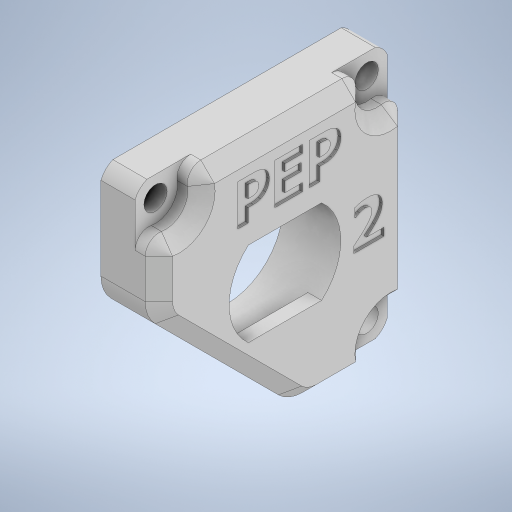
# Autodesk Inventor part: X-Axis-Motor-Support v0.1
Saved by Autodesk Inventor 2023 (Build 270158000, 158)
## iProperties
Created: 2023-07-26
Part Number: X-Axis-Motor-Support v0.1
Material: Generic
Document SubType Name: Modeling
Designer: Parker
Density: 1 g/cm^3
Appearance: Default
Author: Parker
Autodesk Inventor part; units mm, degrees
ref_plane "YZ Plane" through (0, 0, 0) normal (1, 0, 0) x (0, 1, 0)
ref_plane "XZ Plane" through (0, 0, 0) normal (0, 1, 0) x (-1, 0, 0)
ref_plane "XY Plane" through (0, 0, 0) normal (0, 0, 1) x (1, 0, 0)
sketch "Sketch1" plane through (0, 0, 0) normal (1, 0, 0) x (0, 1, 0)
  circle A0 centre (0, 0) radius 8 construction
  circle A1 centre (0, 0) radius 8.2
  line L0 (-15.5, 15.5) -> (15.5, 15.5) construction
  line L1 (15.5, 15.5) -> (15.5, -15.5) construction
  line L2 (15.5, -15.5) -> (-15.5, -15.5) construction
  line L3 (-15.5, -15.5) -> (-15.5, 15.5) construction
  line L4 (-15.5, 15.5) -> (15.5, -15.5) construction
  line L5 (15.5, 15.5) -> (-15.5, -15.5) construction
  line L6 (-18.5, 18.5) -> (18.5, 18.5)
  line L7 (18.5, 18.5) -> (18.5, -18.5)
  line L8 (18.5, -18.5) -> (-18.5, -18.5)
  line L9 (-18.5, -18.5) -> (-18.5, 18.5)
  line L10 (-18.5, 18.5) -> (18.5, -18.5) construction
  line L11 (18.5, 18.5) -> (-18.5, -18.5) construction
  line L12 (-18.5, -2.5) -> (2.5, 18.5)
  point P0 (-15.5, -15.5)
  dimension "d0" = 16
  dimension "d1" = 0.2
  dimension "d2" = 31
  dimension "d3" = 31
  dimension "d4" = 3
  dimension "d5" = 3
  dimension "d6" = 16
  constraints: 26 end point, 5 coincident, 5 parallel, 4 midpoint, 2 centre point, 2 horizontal, 2 perpendicular, 2 point on line
  measures "d0" diameter of A0
  measures "d1" radial gap between concentric circles of A0 A1
  measures "d2" distance of L0.end L1.end
  measures "d3" distance of L0.start L0.end
  measures "d4" distance from line of L8 L1.end
  measures "d5" distance between parallel lines of L7 L1
  measures "d6" distance of L6.end L12.end
extrude "Extrusion1" add sketch "Sketch1" along normal blind 6.5 contours L6 L7 L8 L9 L12
sketch "Sketch2" plane through (6.5, 0, 0) normal (1, 0, 0) x (0, 0, -1)
  point P0 (0, 0)
  point P1 (-15.5, 15.5)
  point P2 (15.5, 15.5)
  point P3 (15.5, -15.5)
hole "Hole1" at (6.5, 15.5, 15.5) at (6.5, 15.5, -15.5) at (6.5, -15.5, -15.5) direction (-1, 0, 0) diameter 3.4 end through all counterbore diameter 6.5 counterbore depth 1.5 clearance for "Socket Head Cap Screw" size "M3" standard "Ansi Metric M Profile"
sketch "Sketch3" plane through (6.5, 0, 0) normal (1, 0, 0) x (0, 0, -1)
  arc A0 (-16.75, 18.5) -> (-18.5, 16.75) centre (-15.5, 15.5) ccw projected
  line L0 (-16.75, 18.5) -> (-18.5, 18.5) projected
  line L1 (-18.5, 18.5) -> (-18.5, 16.75) projected
  arc A1 (18.5, 16.75) -> (16.75, 18.5) centre (15.5, 15.5) ccw projected
  line L2 (18.5, 16.75) -> (18.5, 18.5) projected
  line L3 (18.5, 18.5) -> (16.75, 18.5) projected
  arc A2 (16.75, -18.5) -> (18.5, -16.75) centre (15.5, -15.5) ccw projected
  line L4 (16.75, -18.5) -> (18.5, -18.5) projected
  line L5 (18.5, -18.5) -> (18.5, -16.75) projected
  point P0 (0, 0)
extrude "Extrusion2" cut sketch "Sketch3" against normal through all
fillet "Fillet1" radius 2 6 edges at (5.75, 14.25, 18.5) (5.75, 18.5, 14.25) (5.75, 18.5, -14.25) (5.75, 14.25, -18.5) (5.75, -14.25, -18.5) (5.75, -18.5, -14.25)
fillet "Fillet2" radius 5 2 edges at (3.25, 2.5, 18.5) (3.25, -18.5, -2.5)
sketch "Sketch4" plane through (6.5, 0, 0) normal (1, 0, 0) x (0, 0, -1)
  circle A0 centre (0, 0) radius 8.2 projected
  arc A1 (1.0355, -17.0355) -> (4.5711, -18.5) centre (4.5711, -13.5) ccw projected
  line L0 (4.5711, -18.5) -> (10.3461, -18.5) projected
  arc A2 (10.3461, -18.5) -> (12.3095, -16.119) centre (10.3461, -16.5) ccw projected
  arc A3 (16.119, -12.3095) -> (12.3095, -16.119) centre (15.5, -15.5) ccw projected
  arc A4 (16.119, -12.3095) -> (18.5, -10.3461) centre (16.5, -10.3461) ccw projected
  line L1 (18.5, -10.3461) -> (18.5, 10.3461) projected
  arc A5 (18.5, 10.3461) -> (16.119, 12.3095) centre (16.5, 10.3461) ccw projected
  arc A6 (12.3095, 16.119) -> (16.119, 12.3095) centre (15.5, 15.5) ccw projected
  arc A7 (12.3095, 16.119) -> (10.3461, 18.5) centre (10.3461, 16.5) ccw projected
  line L2 (10.3461, 18.5) -> (-10.3461, 18.5) projected
  arc A8 (-10.3461, 18.5) -> (-12.3095, 16.119) centre (-10.3461, 16.5) ccw projected
  arc A9 (-16.119, 12.3095) -> (-12.3095, 16.119) centre (-15.5, 15.5) ccw projected
  arc A10 (-16.119, 12.3095) -> (-18.5, 10.3461) centre (-16.5, 10.3461) ccw projected
  line L3 (-18.5, 10.3461) -> (-18.5, 4.5711) projected
  arc A11 (-18.5, 4.5711) -> (-17.0355, 1.0355) centre (-13.5, 4.5711) ccw projected
  line L4 (-17.0355, 1.0355) -> (1.0355, -17.0355) projected
  line L5 (-7.5, 10.2) -> (7.5, 10.2)
  line L6 (7.5, 10.2) -> (7.5, 6.2)
  line L7 (7.5, 6.2) -> (-7.5, 6.2)
  line L8 (-7.5, 6.2) -> (-7.5, 10.2)
  circle A12 centre (0, 0) radius 8.2 projected
  line L9 (-7.5, 10.2) -> (7.5, 6.2) construction
  line L10 (7.5, 10.2) -> (-7.5, 6.2) construction
  line L11 (-7.5, -6.2) -> (7.5, -6.2)
  line L12 (7.5, -6.2) -> (7.5, -10.2)
  line L13 (7.5, -10.2) -> (-7.5, -10.2)
  line L14 (-7.5, -10.2) -> (-7.5, -6.2)
  line L15 (-7.5, -6.2) -> (7.5, -10.2) construction
  line L16 (7.5, -6.2) -> (-7.5, -10.2) construction
  point P0 (0, 8.2)
  point P1 (0, -8.2)
  point P2 (-7.5, -8.5)
  point P3 (-5.8, -10.2)
  point P4 (-5.3666, -6.2)
  point P5 (-5.3666, 6.2)
  point P6 (5.3666, 6.2)
  point P7 (5.3666, -6.2)
  dimension "d20" = 15
  dimension "d21" = 4
  dimension "d22" = 15
  dimension "d23" = 4
  constraints: 24 end point, 4 midpoint, 4 parallel, 2 horizontal, 2 perpendicular, 2 point on circle
  measures "d20" distance of L6.end L7.end
  measures "d21" distance of L5.end L6.end
  measures "d22" distance of L12.end L13.end
  measures "d23" distance of L11.end L12.end
extrude "Extrusion3" add sketch "Sketch4" along normal blind 2 contours A0 L7 L6 L5 L8 L11 L14 L4 A11 L3 A10 A9 A8 L2 A7 A6 A5 L1 A4 A3 A2 L0 A1 L13 L12 | L7 A0 | A0 L7 L8 L5 L6 | L11 L12 L13 L4 L14 A0 | A0 L11
chamfer "Chamfer2" distance 2 angle 45 16 edges at (8.5, 18.5, 0) (8.5, 17.7724, 11.8892) (8.5, 13.2019, 13.2019) (8.5, 11.8892, 17.7724) (8.5, 7.4586, 18.5) (8.5, 2.6577, 18.1194) (8.5, -8, 8) (8.5, -18.1194, -2.6577) (8.5, -18.5, -7.4586) (8.5, -17.7724, -11.8892) (8.5, -13.2019, -13.2019) (8.5, -11.8892, -17.7724) (8.5, 0, -18.5) (8.5, 11.8892, -17.7724) (8.5, 13.2019, -13.2019) (8.5, 17.7724, -11.8892)
sketch "Sketch5" plane through (8.5, 0, 0) normal (1, 0, 0) x (0, 0, -1)
  line L0 (9.5104, 3.5032) -> (16.5185, 3.5032) construction
  line L1 (16.5185, 3.5032) -> (16.5185, -4.6524) construction
  line L2 (16.5185, -4.6524) -> (9.5104, -4.6524) construction
  line L3 (9.5104, -4.6524) -> (9.5104, 3.5032) construction
  line L4 (-7.5472, 15.0221) -> (-0.5391, 15.0221) construction
  line L5 (-0.5391, 15.0221) -> (-0.5391, 6.8665) construction
  line L6 (-0.5391, 6.8665) -> (-7.5472, 6.8665) construction
  line L7 (-7.5472, 6.8665) -> (-7.5472, 15.0221) construction
  line L8 (14.5282, -2.6135) -> (10.1182, -2.6135)
  line L9 (10.1182, -2.6135) -> (10.1182, -1.6362)
  spline S0 degree 2 poles (10.1182, -1.6362) (10.6773, -1.1889) (11.572, -0.4012) (11.9075, -0.0463) knots 0 0 0 1 2 2 2
  spline S1 degree 2 poles (11.9075, -0.0463) (12.3499, 0.4156) (12.7438, 1.1207) (12.7438, 1.4902) knots 0 0 0 1 2 2 2
  spline S2 degree 2 poles (12.7438, 1.4902) (12.7438, 1.9083) (12.243, 2.3557) (11.7956, 2.3557) knots 0 0 0 1 2 2 2
  spline S3 degree 2 poles (11.7956, 2.3557) (11.5671, 2.3557) (11.1587, 2.2438) (10.9496, 2.1563) knots 0 0 0 1 2 2 2
  spline S4 degree 2 poles (10.9496, 2.1563) (10.7454, 2.0639) (10.4537, 1.8694) (10.3807, 1.8208) knots 0 0 0 1 2 2 2
  line L10 (10.3807, 1.8208) -> (10.264, 1.8208)
  line L11 (10.264, 1.8208) -> (10.264, 3.1288)
  spline S5 degree 2 poles (10.264, 3.1288) (10.5169, 3.2503) (11.5963, 3.5032) (12.0971, 3.5032) knots 0 0 0 1 2 2 2
  spline S6 degree 2 poles (12.0971, 3.5032) (13.1668, 3.5032) (14.2656, 2.5502) (14.2656, 1.6895) knots 0 0 0 1 2 2 2
  spline S7 degree 2 poles (14.2656, 1.6895) (14.2656, 1.1596) (13.7648, 0.1385) (13.1862, -0.445) knots 0 0 0 1 2 2 2
  spline S8 degree 2 poles (13.1862, -0.445) (12.8216, -0.8048) (12.136, -1.3639) (11.9853, -1.4806) knots 0 0 0 1 2 2 2
  line L12 (11.9853, -1.4806) -> (14.5282, -1.4806)
  line L13 (14.5282, -1.4806) -> (14.5282, -2.6135)
  spline S9 degree 2 poles (-2.3106, 13.1307) (-2.3106, 12.7126) (-2.578, 11.9541) (-2.826, 11.7012) knots 0 0 0 1 2 2 2
  spline S10 degree 2 poles (-2.826, 11.7012) (-2.9767, 11.5408) (-3.3462, 11.2782) (-3.565, 11.1858) knots 0 0 0 1 2 2 2
  spline S11 degree 2 poles (-3.565, 11.1858) (-3.7887, 11.0935) (-4.309, 10.9865) (-4.6299, 10.9865) knots 0 0 0 1 2 2 2
  line L14 (-4.6299, 10.9865) -> (-5.4176, 10.9865)
  line L15 (-5.4176, 10.9865) -> (-5.4176, 9.0221)
  line L16 (-5.4176, 9.0221) -> (-6.9249, 9.0221)
  line L17 (-6.9249, 9.0221) -> (-6.9249, 15.0221)
  line L18 (-6.9249, 15.0221) -> (-4.5958, 15.0221)
  spline S12 degree 2 poles (-4.5958, 15.0221) (-4.0804, 15.0221) (-3.3268, 14.8325) (-3.0205, 14.6283) knots 0 0 0 1 2 2 2
  spline S13 degree 2 poles (-3.0205, 14.6283) (-2.6801, 14.3998) (-2.3106, 13.651) (-2.3106, 13.1307) knots 0 0 0 1 2 2 2
  spline S14 degree 2 poles (-3.8568, 13.0918) (-3.8568, 13.3495) (-4.0999, 13.7142) (-4.2652, 13.7823) knots 0 0 0 1 2 2 2
  spline S15 degree 2 poles (-4.2652, 13.7823) (-4.4791, 13.8747) (-4.8681, 13.9038) (-5.2036, 13.9038) knots 0 0 0 1 2 2 2
  line L19 (-5.2036, 13.9038) -> (-5.4176, 13.9038)
  line L20 (-5.4176, 13.9038) -> (-5.4176, 12.1048)
  line L21 (-5.4176, 12.1048) -> (-5.3106, 12.1048)
  spline S16 degree 2 poles (-5.3106, 12.1048) (-5.1015, 12.1048) (-4.7223, 12.1145) (-4.5813, 12.1388) knots 0 0 0 1 2 2 2
  spline S17 degree 2 poles (-4.5813, 12.1388) (-4.4597, 12.1583) (-4.1923, 12.275) (-4.1193, 12.3479) knots 0 0 0 1 2 2 2
  spline S18 degree 2 poles (-4.1193, 12.3479) (-3.9637, 12.4938) (-3.8568, 12.8195) (-3.8568, 13.0918) knots 0 0 0 1 2 2 2
  line L22 (-1.5035, 9.0221) -> (-1.5035, 15.0221)
  line L23 (-1.5035, 15.0221) -> (2.5516, 15.0221)
  line L24 (2.5516, 15.0221) -> (2.5516, 13.8795)
  line L25 (2.5516, 13.8795) -> (-0.0059, 13.8795)
  line L26 (-0.0059, 13.8795) -> (-0.0059, 12.8244)
  line L27 (-0.0059, 12.8244) -> (2.3523, 12.8244)
  line L28 (2.3523, 12.8244) -> (2.3523, 11.6818)
  line L29 (2.3523, 11.6818) -> (-0.0059, 11.6818)
  line L30 (-0.0059, 11.6818) -> (-0.0059, 10.1648)
  line L31 (-0.0059, 10.1648) -> (2.5516, 10.1648)
  line L32 (2.5516, 10.1648) -> (2.5516, 9.0221)
  line L33 (2.5516, 9.0221) -> (-1.5035, 9.0221)
  spline S19 degree 2 poles (8.187, 13.1307) (8.187, 12.7126) (7.9196, 11.9541) (7.6716, 11.7012) knots 0 0 0 1 2 2 2
  spline S20 degree 2 poles (7.6716, 11.7012) (7.5209, 11.5408) (7.1513, 11.2782) (6.9325, 11.1858) knots 0 0 0 1 2 2 2
  spline S21 degree 2 poles (6.9325, 11.1858) (6.7089, 11.0935) (6.1886, 10.9865) (5.8677, 10.9865) knots 0 0 0 1 2 2 2
  line L34 (5.8677, 10.9865) -> (5.08, 10.9865)
  line L35 (5.08, 10.9865) -> (5.08, 9.0221)
  line L36 (5.08, 9.0221) -> (3.5727, 9.0221)
  line L37 (3.5727, 9.0221) -> (3.5727, 15.0221)
  line L38 (3.5727, 15.0221) -> (5.9017, 15.0221)
  spline S22 degree 2 poles (5.9017, 15.0221) (6.4171, 15.0221) (7.1708, 14.8325) (7.4771, 14.6283) knots 0 0 0 1 2 2 2
  spline S23 degree 2 poles (7.4771, 14.6283) (7.8175, 14.3998) (8.187, 13.651) (8.187, 13.1307) knots 0 0 0 1 2 2 2
  spline S24 degree 2 poles (6.6408, 13.0918) (6.6408, 13.3495) (6.3977, 13.7142) (6.2324, 13.7823) knots 0 0 0 1 2 2 2
  spline S25 degree 2 poles (6.2324, 13.7823) (6.0184, 13.8747) (5.6294, 13.9038) (5.2939, 13.9038) knots 0 0 0 1 2 2 2
  line L39 (5.2939, 13.9038) -> (5.08, 13.9038)
  line L40 (5.08, 13.9038) -> (5.08, 12.1048)
  line L41 (5.08, 12.1048) -> (5.187, 12.1048)
  spline S26 degree 2 poles (5.187, 12.1048) (5.3961, 12.1048) (5.7753, 12.1145) (5.9163, 12.1388) knots 0 0 0 1 2 2 2
  spline S27 degree 2 poles (5.9163, 12.1388) (6.0379, 12.1583) (6.3053, 12.275) (6.3782, 12.3479) knots 0 0 0 1 2 2 2
  spline S28 degree 2 poles (6.3782, 12.3479) (6.5338, 12.4938) (6.6408, 12.8195) (6.6408, 13.0918) knots 0 0 0 1 2 2 2
  point P0 (0, 0)
  constraints: 4 other
extrude "Extrusion4" cut sketch "Sketch5" against normal blind 0.4
body "Solid1"
